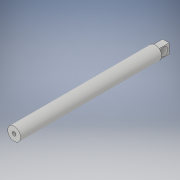
# Autodesk Inventor part: SolenoidCase
Saved by Autodesk Inventor 2018 (Build 220112000, 112)
## iProperties
Created: 2018-05-31
Part Number: SolenoidCase
Material: Generic
Document SubType Name: Modeling
Designer: choices
Density: 1 g/cm^3
Appearance: Default
Author: choices
Autodesk Inventor part; units mm, degrees
ref_plane "YZ Plane" through (0, 0, 0) normal (1, 0, 0) x (0, 1, 0)
ref_plane "XZ Plane" through (0, 0, 0) normal (0, 1, 0) x (-1, 0, 0)
ref_plane "XY Plane" through (0, 0, 0) normal (0, 0, 1) x (1, 0, 0)
sketch "Sketch1" plane through (0, 0, 0) normal (0, 0, 1) x (1, 0, 0)
  line L0 (0, 0) -> (10.16, 0)
  line L1 (10.16, 0) -> (10.16, 15.24)
  line L2 (10.16, 15.24) -> (0, 15.24)
  line L3 (0, 15.24) -> (0, 0)
  dimension "d0" = 10.16
  dimension "d1" = 15.24
  constraints: 8 end point, 2 parallel, 1 horizontal, 1 perpendicular
  measures "d0" distance of L2.end L1.end
  measures "d1" distance of L1.end L0.end
extrude "Extrusion1" add sketch "Sketch1" along normal blind 16.51
sketch "Sketch2" plane through (10.16, 0, 0) normal (1, 0, 0) x (0, 0, -1)
  circle A0 centre (-8.255, 7.62) radius 6.35
  line L0 (0, 15.24) -> (-16.51, 15.24) projected
  point P0 (0, 0)
  dimension "d4" = 12.7
  dimension "d5" = 7.62
  constraints: 1 centre point
  measures "d4" diameter of A0
  measures "d5" distance from line of L0 A0.centre
extrude "Extrusion2" cut sketch "Sketch2" against normal blind 16.51
sketch "Sketch3" plane through (0, 0, 16.51) normal (0, 0, 1) x (1, 0, 0)
  circle A0 centre (5.08, 8.152) radius 10.16
  point P0 (0, 0)
  dimension "d8" = 20.32
  constraints: 1 centre point
  measures "d8" diameter of A0
extrude "Extrusion3" add sketch "Sketch3" along normal blind 219.075
sketch "Sketch5" plane through (5.08, 8.152, 235.585) normal (0, 0, 1) x (1, 0, 0)
  circle A0 centre (0, 0) radius 2.921
  point P0 (-5.08, -8.152)
  dimension "d13" = 5.842
  constraints: 1 centre point
  measures "d13" diameter of A0
extrude "Extrusion5" cut sketch "Sketch5" against normal blind 152.4
body "Solid1"
